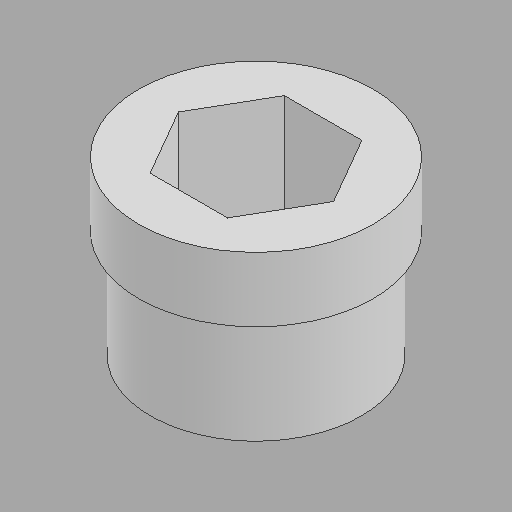
# Autodesk Inventor part: WHEEL_ADAPTER
Saved by Autodesk Inventor 2025.2 (Build 292293000, 293)
## iProperties
Created: 2026-06-27
Part Number: WHEEL_ADAPTER
Material: Generic
Document SubType Name: Modeling
Designer: Ben
Density: 1 g/cm^3
Appearance: Default
Author: Ben
Autodesk Inventor part; units mm, degrees
ref_plane "YZ Plane" through (0, 0, 0) normal (1, 0, 0) x (0, 1, 0)
ref_plane "XZ Plane" through (0, 0, 0) normal (0, 1, 0) x (-1, 0, 0)
ref_plane "XY Plane" through (0, 0, 0) normal (0, 0, 1) x (1, 0, 0)
sketch "Sketch2" plane through (0, 0, 0) normal (0, 0, 1) x (1, 0, 0)
  line L0 (0, 0) -> (10.9, 0)
  line L1 (10.9, 0) -> (10.9, 6)
  line L2 (10.9, 6) -> (0, 6)
  line L3 (0, 6) -> (0, 0)
  line L4 (0, 0) -> (9.8, 0)
  line L5 (9.8, 0) -> (9.8, -10)
  line L6 (9.8, -10) -> (0, -10)
  line L7 (0, -10) -> (0, 0)
  dimension "d1" = 10.9
  dimension "d2" = 6
  dimension "d3" = 9.8
  dimension "d4" = 10
  constraints: 16 end point, 4 parallel, 2 horizontal, 2 perpendicular
  measures "d1" distance of L1.end L2.end
  measures "d2" distance of L0.end L1.end
  measures "d3" distance of L5.end L6.end
  measures "d4" distance of L4.end L5.end
revolve "Revolution1" add sketch "Sketch2" angle 360 about axis through (0, 6, 0) along (0, -1, 0)
sketch "Sketch5" plane through (0, 6, 0) normal (0, 1, 0) x (1, 0, 0)
  line L0 (3.6084, 6.25) -> (7.2169, 0)
  line L1 (7.2169, 0) -> (3.6084, -6.25)
  line L2 (3.6084, -6.25) -> (-3.6084, -6.25)
  line L3 (-3.6084, -6.25) -> (-7.2169, 0)
  line L4 (-7.2169, 0) -> (-3.6084, 6.25)
  line L5 (-3.6084, 6.25) -> (3.6084, 6.25)
  point P0 (0, 0)
  point P1 (0, 0)
  dimension "d16" = 12.5
  constraints: 12 end point, 1 coincident, 1 horizontal alignment, 13 other
  measures "d16" distance between parallel lines of L2 L5
extrude "Extrusion2" cut sketch "Sketch5" against normal blind 14
sketch "Sketch6" plane through (0, -10, 0) normal (0, -1, 0) x (1, 0, 0)
  circle A0 centre (0, 0) radius 2.5
  point P0 (0, 0)
  dimension "d19" = 5
  constraints: 1 centre point, 1 coincident
  measures "d19" diameter of A0
extrude "Extrusion3" cut sketch "Sketch6" against normal through all
body "Solid1"
